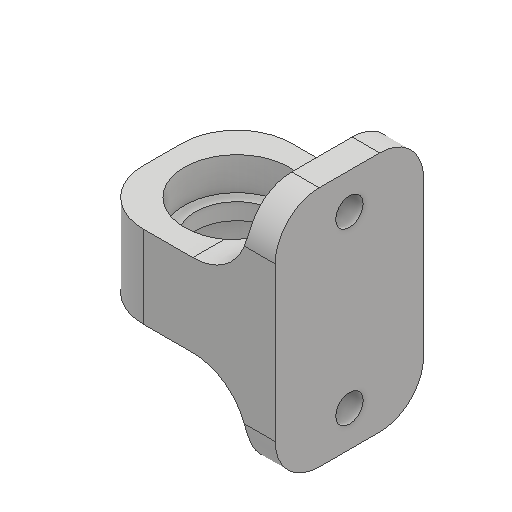
# Autodesk Inventor part: 3DP_ABS_Y_Axis_Pulley_Rod_Mid_Bearing_Block
Saved by Autodesk Inventor 2026.1 (Build 301233000, 233)
## iProperties
Created: 2016-06-19
Part Number: 3DP_ABS_Y_Axis_Pulley_Rod_Mid_Bearing_Block
Material: Ogólny
Document SubType Name: Modeling
Designer: Andrzej
Density: 1 g/cm^3
Appearance: Domyślna
Mass: 13.6975 g
Surface Area: 56.2187 cm^2
Volume: 13.6975 cm^3
Author: Andrzej
Autodesk Inventor part; units mm, degrees
ref_plane "YZ Plane" through (0, 0, 0) normal (1, 0, 0) x (0, 1, 0)
ref_plane "XZ Plane" through (0, 0, 0) normal (0, 1, 0) x (-1, 0, 0)
ref_plane "XY Plane" through (0, 0, 0) normal (0, 0, 1) x (1, 0, 0)
sketch "Szkic1" plane through (0, 0, 0) normal (0, 0, 1) x (1, 0, 0)
  line L0 (-15.5705, 13.388) -> (18.4295, 13.388)
  line L1 (18.4295, 13.388) -> (18.4295, -13.612)
  line L2 (18.4295, -13.612) -> (-15.5705, -13.612)
  line L3 (-15.5705, -13.612) -> (-15.5705, 13.388)
  circle A0 centre (-2.0705, -0.112) radius 9.5
  point P0 (0, 0)
  dimension "d0" = 27
  dimension "d1" = 34
  dimension "d2" = 20.5
  dimension "d3" = 13.5
  dimension "d4" = 19
  constraints: 8 end point, 2 parallel, 1 centre point, 1 coincident, 1 horizontal, 1 perpendicular
  measures "d0" distance of L0.end L1.end
  measures "d1" distance of L1.end L2.end
  measures "d2" distance from line of L1 point (-2.071, -0.112)
  measures "d3" distance from line of point (-2.071, -0.112) L0
  measures "d4" diameter of A0
extrude "Wyciągnięcie proste1" add sketch "Szkic1" along normal blind 15 contours L0 L1 L2 L3 | A0
extrude "Wyciągnięcie proste2" cut sketch "Szkic1" along normal blind 6 contours A0
sketch "Szkic2" plane through (0, 0, 15) normal (0, 0, 1) x (1, 0, 0)
  circle A0 centre (-2.0705, -0.112) radius 9.5 projected
  line L0 (18.4295, 13.388) -> (-15.5705, 13.388) projected
  line L1 (-15.5705, 13.388) -> (-15.5705, -13.612) projected
  line L2 (-15.5705, -13.612) -> (18.4295, -13.612) projected
  line L3 (18.4295, -13.612) -> (18.4295, 13.388) projected
  point P0 (0, 0)
extrude "Wyciągnięcie proste3" cut sketch "Szkic2" against normal blind 6 contours A0
hole "Otwór1" at (-2.0705, -0.112, 0) direction (0, 0, 1) diameter 15 end through all
fillet "Zaokrąglenie1" radius 10 2 edges at (-15.5705, 13.388, 7.5) (-15.5705, -13.612, 7.5)
sketch "Szkic3" plane through (18.4295, -13.612, 0) normal (1, 0, 0) x (0, 0, -1)
  line L0 (0, 27) -> (0, 0) projected
  line L1 (0, 27) -> (-15, 27) projected
  line L2 (-15, 0) -> (-15, 27) projected
  line L3 (0, 0) -> (-15, 0) projected
  line L4 (-15, 27) -> (-29.5, 27)
  line L5 (-29.5, 27) -> (-29.5, 0)
  line L6 (-29.5, 0) -> (-15, 0)
  line L7 (0, 27) -> (14.5, 27)
  line L8 (14.5, 27) -> (14.5, 0)
  line L9 (14.5, 0) -> (0, 0)
  point P0 (0, 13.612)
  point P1 (-23, 13.5)
  point P2 (8, 13.5)
  dimension "d21" = 14.5
  dimension "d22" = 14.5
  dimension "d23" = 6.5
  dimension "d24" = 6.5
  dimension "d25" = 27
  dimension "d26" = 13.5
  dimension "d27" = 13.5
  constraints: 12 end point, 3 perpendicular, 1 horizontal, 1 point on line, 1 vertical
  measures "d21" distance of L1.end L4.end
  measures "d22" distance of L0.start L7.end
  measures "d23" distance from line of L5 point (-23, 13.5)
  measures "d24" distance from line of L8 point (8, 13.5)
  measures "d25" distance of L4.end L5.end
  measures "d26" distance from line of L4 point (-23, 13.5)
  measures "d27" distance from line of L7 point (8, 13.5)
extrude "Wyciągnięcie proste4" add sketch "Szkic3" against normal blind 5 contours L7 L8 L9 L0 | L2 L6 L5 L4
hole "Otwór2" at (18.4295, -0.112, 23) at (18.4295, -0.112, -8) direction (-1, 0, 0) diameter 5 end through all
fillet "Zaokrąglenie2" radius 10 2 edges at (13.4295, -0.112, 15) (13.4295, -0.112, 0)
fillet "Zaokrąglenie3" radius 8 4 edges at (15.9295, 13.388, -14.5) (15.9295, -13.612, -14.5) (15.9295, -13.612, 29.5) (15.9295, 13.388, 29.5)
sketch "Szkic4" plane through (13.4295, -13.612, 0) normal (-1, 0, 0) x (0, 0, 1)
  arc A0 (-10, 15) -> (-10, 12) centre (-8, 13.5) ccw projected
  arc A1 (25, 12) -> (25, 15) centre (23, 13.5) ccw projected
  circle A2 centre (-8, 13.5) radius 5
  circle A3 centre (23, 13.5) radius 5
  point P0 (0, 13.612)
  dimension "d37" = 10
  dimension "d38" = 10
  constraints: 2 centre point, 2 coincident
  measures "d37" diameter of A2
  measures "d38" diameter of A3
extrude "Wyciągnięcie proste5" cut sketch "Szkic4" along normal blind 5
equation "\"d3\" = 0.5 * d0"
equation "\"d24\" = d23"
equation "\"d26\" = 0.5 * d25"
equation "\"d27\" = d26"
